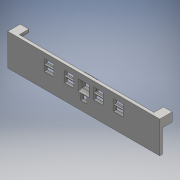
# Autodesk Inventor part: bottom-test
Saved by Autodesk Inventor 2016 (Build 200138000, 138)
## iProperties
Created: 2016-04-02
Part Number: bottom-test
Material: Generic
Document SubType Name: Modeling
Designer: jferner
Density: 1 g/cm^3
Appearance: Default
Author: jferner
Autodesk Inventor part; units mm, degrees
ref_plane "YZ Plane" through (0, 0, 0) normal (1, 0, 0) x (0, 1, 0)
ref_plane "XZ Plane" through (0, 0, 0) normal (0, 1, 0) x (-1, 0, 0)
ref_plane "XY Plane" through (0, 0, 0) normal (0, 0, 1) x (1, 0, 0)
sketch "Sketch1" plane through (0, 0, 0) normal (0, 1, 0) x (-1, 0, 0)
  line L0 (0, 0) -> (-52.5, 0)
  line L1 (-52.5, 0) -> (-52.5, 11)
  line L2 (-52.5, 11) -> (0, 11)
  line L3 (0, 11) -> (0, 0)
  dimension "d0" = 52.5
  dimension "d1" = 11
  constraints: 8 end point, 2 parallel, 1 horizontal, 1 perpendicular
  measures "d0" distance of L1.end L2.end
  measures "d1" distance of L0.end L1.end
extrude "Extrusion1" add sketch "Sketch1" along normal blind 1
sketch "Sketch6" plane through (0, 1, 0) normal (0, 1, 0) x (1, 0, 0)
  line L0 (0, -11) -> (52.5, -11) projected
  line L1 (0, 0) -> (1, 0)
  line L2 (1, -8) -> (1, -10)
  line L3 (1.5543, -11) -> (0, -11)
  line L4 (0, -11) -> (0, 0)
  line L5 (52.5, -11) -> (52.5, 0) projected
  line L6 (0, -11) -> (52.5, -11)
  line L7 (52.5, -11) -> (52.5, -9.2245)
  line L8 (0, -9.2245) -> (0, -11)
  line L9 (52.5, -11) -> (49.8731, -11)
  line L10 (51.5, -10) -> (51.5, -8)
  line L11 (51, 0) -> (52.5, 0)
  line L12 (52.5, 0) -> (52.5, -11)
  line L13 (52.5, -8) -> (51.5, -8)
  line L14 (49.5, -10) -> (49.5, -11)
  line L15 (3, -11) -> (3, -10)
  line L16 (1, -8) -> (0, -8)
  line L17 (51.5, -10) -> (49.5, -10)
  line L18 (3, -10) -> (1, -10)
  dimension "d41" = 1
  dimension "d43" = 1
  dimension "d83" = 2
  dimension "d85" = 2
  constraints: 34 end point, 9 point on line, 8 parallel, 5 perpendicular, 3 horizontal
  measures "d41" distance between parallel lines of L4 L2
  measures "d43" distance between parallel lines of L5 L10
  measures "d83" distance between parallel lines of L10 L14
  measures "d85" distance between parallel lines of L2 L15
extrude "walls" add sketch "Sketch6" along normal blind 3.3
sketch "Sketch2" plane through (0, 1, 0) normal (0, 1, 0) x (1, 0, 0)
  circle A0 centre (4, -5) radius 1.5
  circle A1 centre (48.5, -5) radius 1.5
  line L0 (52.5, -11) -> (52.5, 0) projected
  line L1 (0, 0) -> (0, -11) projected
  line L2 (52.5, 0) -> (0, 0) projected
  line L3 (1, -10) -> (1, -8) projected
  line L4 (51.5, -8) -> (51.5, -10) projected
  point P0 (1, 0)
  point P1 (51, 0)
  dimension "d5" = 3
  dimension "d8" = 5
  dimension "d46" = 3
  dimension "d47" = 3
  constraints: 2 centre point, 1 equal radius, 1 horizontal alignment, 1 other
  measures "d5" diameter of A1
  measures "d8" distance from line of L2 A0.centre
  measures "d46" distance from line of L3 A0.centre
extrude "Extrusion2" add sketch "Sketch2" along normal blind 1.6
sketch "Sketch3" plane through (0, 0, 0) normal (0, -1, 0) x (1, 0, 0)
  line L0 (12.7, 9.2) -> (15.9, 9.2)
  line L1 (15.9, 9.2) -> (15.9, 7.5)
  line L2 (15.9, 7.5) -> (12.7, 7.5)
  line L3 (12.7, 7.5) -> (12.7, 9.2)
  line L4 (12.7, 7.1) -> (15.9, 7.1)
  line L5 (15.9, 7.1) -> (15.9, 5.4)
  line L6 (15.9, 5.4) -> (12.7, 5.4)
  line L7 (12.7, 5.4) -> (12.7, 7.1)
  line L8 (0, 11) -> (0, 0) projected
  line L9 (0, 0) -> (52.5, 0) projected
  line L10 (1, 10) -> (1, 8) projected
  line L11 (1, 10) -> (51.5, 10) projected
  point P0 (1, 0)
  dimension "d12" = 3.2
  dimension "d15" = 1.7
  dimension "d16" = 1.7
  dimension "d17" = 0.4
  dimension "d48" = 11.7
  dimension "d69" = 0.8
  constraints: 16 end point, 4 parallel, 2 horizontal, 2 perpendicular, 2 point on line
  measures "d12" distance of L0.start L0.end
  measures "d15" distance of L2.end L0.start
  measures "d16" distance of L6.end L4.start
  measures "d17" distance between parallel lines of L4 L2
  measures "d48" distance between parallel lines of L10 L3
  measures "d69" distance between parallel lines of L0 L11
extrude "lineSensorHole" cut sketch "Sketch3" against normal through all
chamfer "Chamfer2" distance 0.5 angle 10 1 edges at (14.3, 0, 7.5) measured on face at (14.8333, 0.3333, 7.5)
chamfer "Chamfer3" distance 0.5 angle 10 1 edges at (14.3, 0, 7.1) measured on face at (13.7667, 0.3333, 7.1)
pattern_linear "Rectangular Pattern3" count 2 spacing 6.95 along (1, 0, 0) of "lineSensorHole", "Chamfer2", "Chamfer3"
sketch "Sketch4" plane through (0, 0, 0) normal (0, -1, 0) x (1, 0, 0)
  line L0 (24.375, 9) -> (28.125, 9)
  line L1 (28.125, 9) -> (28.125, 5.63)
  line L2 (28.125, 5.63) -> (24.375, 5.63)
  line L3 (24.375, 5.63) -> (24.375, 9)
  line L4 (0, 11) -> (0, 0) projected
  line L5 (0, 0) -> (52.5, 0) projected
  line L6 (25.25, 5.06) -> (27.25, 5.06)
  line L7 (27.25, 5.06) -> (27.25, 3.02)
  line L8 (27.25, 3.02) -> (25.25, 3.02)
  line L9 (25.25, 3.02) -> (25.25, 5.06)
  line L10 (1, 10) -> (1, 8) projected
  line L11 (1, 10) -> (51.5, 10) projected
  line L12 (31.8053, 3.52) -> (28.9848, 3.52)
  line L13 (31.8053, 4.56) -> (28.9848, 4.56)
  line L14 (31.8053, 6.13) -> (28.9848, 6.13)
  line L15 (28.9848, 8.5) -> (31.8053, 8.5)
  point P0 (1, 0)
  dimension "colorSensorWindowWidth" = 3.75
  dimension "ledWindowWidth" = 2
  dimension "d34" = 0.875
  dimension "d49" = 23.375
  dimension "d86" = 6.48
  dimension "d87" = 5.44
  dimension "d88" = 3.87
  dimension "d89" = 1.5
  dimension "d90" = 0.5
  dimension "d91" = 0.5
  dimension "d92" = 0.5
  dimension "d93" = 0.5
  constraints: 24 end point, 6 horizontal, 4 parallel, 4 vertical alignment, 2 perpendicular
  measures "colorSensorWindowWidth" distance of L0.start L0.end
  measures "ledWindowWidth" distance of L6.start L6.end
  measures "d34" distance between parallel lines of L1 L7
  measures "d49" distance between parallel lines of L10 L3
  measures "d86" distance between parallel lines of L11 L12
  measures "d87" distance between parallel lines of L11 L13
  measures "d88" distance between parallel lines of L11 L14
  measures "d89" distance between parallel lines of L11 L15
  measures "d90" distance between parallel lines of L14 L2
  measures "d91" distance between parallel lines of L15 L0
  measures "d92" distance between parallel lines of L13 L6
  measures "d93" distance between parallel lines of L12 L8
extrude "colorSensorHole" cut sketch "Sketch4" against normal through all
sketch "Sketch5" plane through (0, 1, 0) normal (0, 1, 0) x (1, 0, 0)
  line L0 (23.875, -5.13) -> (28.625, -5.13)
  line L1 (28.625, -5.13) -> (28.625, -9.5)
  line L2 (28.625, -9.5) -> (23.875, -9.5)
  line L3 (23.875, -9.5) -> (23.875, -5.13)
  line L4 (28.125, -9) -> (24.375, -9) projected
  line L5 (28.125, -5.63) -> (28.125, -9) projected
  line L6 (24.375, -5.63) -> (28.125, -5.63) projected
  line L7 (24.375, -9) -> (24.375, -5.63) projected
  point P0 (0, 0)
  dimension "d35" = 0.5
  dimension "d36" = 0.5
  dimension "d37" = 0.5
  dimension "d38" = 0.5
  constraints: 8 end point, 2 parallel, 1 horizontal, 1 perpendicular
  measures "d35" distance between parallel lines of L4 L2
  measures "d36" distance between parallel lines of L5 L1
  measures "d37" distance between parallel lines of L0 L6
  measures "d38" distance between parallel lines of L3 L7
extrude "Extrusion5" add sketch "Sketch5" along normal blind 1.6
pattern_linear "Rectangular Pattern4" count 2 spacing 17 along (1, 0, 0) of "lineSensorHole", "Chamfer2", "Chamfer3", "Rectangular Pattern3"
chamfer "Chamfer4" distance 1.4 angle 15 1 edges at (26.25, 0, 5.63) measured on face at (25.625, 0.8667, 5.63)
equation "\"d0\" = pcbWidthWithTolerance + 2 * wallThickness"
equation "\"d41\" = wallThickness"
equation "\"d43\" = wallThickness"
equation "\"d63\" = lineSensorChamferDepth"
equation "\"d65\" = lineSensorChamferAngle"
equation "\"d34\" = -0.5 * ledWindowWidth + 0.5 * colorSensorWindowWidth"
equation "\"d49\" = -0.5 * colorSensorWindowWidth + 0.5 * pcbWidthWithTolerance"
equation "\"d39\" = heightFromPcb"
equation "\"wallThickness\" = 1"
equation "\"pcbWidthWithTolerance\" = 50.5"
equation "\"lineSensorChamferDepth\" = 0.5"
equation "\"lineSensorChamferAngle\" = 10deg"
equation "\"heightFromPcb\" = 1.6"
body "Solid1"
